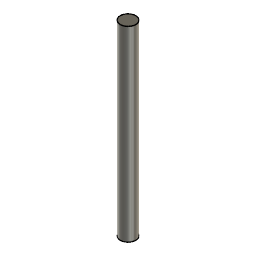
exp6 (Autodesk Fusion 360 archive; units mm, degrees)
design "Base stand attach"
part number: 2026-03-17-14-04-28-907
Autodesk Fusion 360 part; units mm, degrees
sketch "Sketch3" plane through (0, 0, 0) normal (0, 1, 0) x (1, 0, 0)
sketch "Sketch4" plane through (0, 0, 0) normal (0, 0, 1) x (1, 0, 0)
  circle A0 centre (0, 0) radius 1
  dimension "d5" = 2
  constraint coincident A0.centre origin
  measures "d5" diameter of A0
extrude "Extrude2" add sketch "Sketch4" along normal blind 24

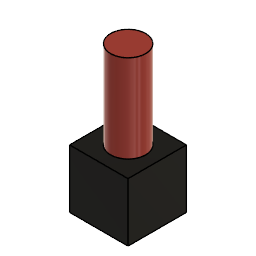
design "Base Box"
part number: 2026-03-16-21-54-47-884
Autodesk Fusion 360 part; units mm, degrees
sketch "Sketch1" plane through (0, 0, 0) normal (0, 0, 1) x (1, 0, 0)
  line L0 (0, 0) -> (10, 0)
  line L1 (10, 0) -> (10, -10)
  line L2 (10, -10) -> (0, -10)
  line L3 (0, -10) -> (0, 0)
  dimension "d1" = 10
  dimension "d2" = 10
  constraint horizontal L0
  constraint vertical L1
  constraint horizontal L2
  constraint vertical L3
  constraint coincident L0.start L3.end
  measures "d1" distance of L0.start L0.end
  measures "d2" distance of L0.start L2.end
extrude "Extrude1" add sketch "Sketch1" along normal blind 10
sketch "Sketch2" plane through (0, 0, 10) normal (0, 0, 1) x (-1, 0, 0)
  line L0 (0, 10) -> (-10, 10)
  line L1 (-10, 10) -> (-10, 0)
  line L2 (-10, 0) -> (0, 0)
  line L3 (0, 0) -> (0, 10)
  circle A0 centre (-5, 4.9796) radius 3
  dimension "d5" = 6
  measures "d5" diameter of A0
extrude "Extrude2" add sketch "Sketch2" along normal blind 15 contours A0

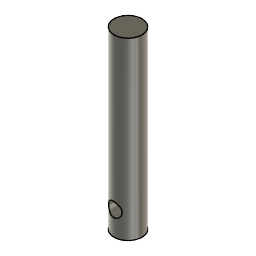
design "Base stand final"
part number: 2026-03-17-13-57-48-070
Autodesk Fusion 360 part; units mm, degrees
sketch "Sketch1" plane through (0, 0, 0) normal (0, 1, 0) x (1, 0, 0)
form "Form1" [no effect]
sketch "sketch 236" plane through (0, 0, 0) normal (0, 0, 1) x (1, 0, 0)
  circle A0 centre (0, 0) radius 2
  constraint coincident A0.centre origin
extrude "Extrude1" add sketch "sketch 236" along normal blind 25
sketch "Sketch2" plane through (0, 0, 0) normal (0, 1, 0) x (1, 0, 0)
  circle A0 centre (-0.0644, -3.4131) radius 1.5
  dimension "d3" = 3
  measures "d3" diameter of A0
hole "Hole1" at (-0.0644, 0, 3.4131) direction (0, -1, 0) diameter 2 depth 2 tip angle 118
